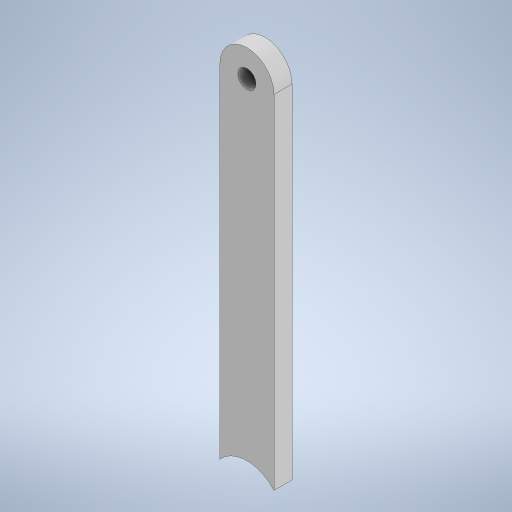
# Autodesk Inventor part: Conn Rod Rod Portion
Saved by Autodesk Inventor 2023 (Build 270158000, 158)
## iProperties
Created: 2023-02-24
Part Number: Conn Rod Rod Portion
Material: Generic
Document SubType Name: Modeling
Designer: tommy
Density: 1 g/cm^3
Appearance: Default
Author: tommy
Autodesk Inventor part; units mm, degrees
ref_plane "YZ Plane" through (0, 0, 0) normal (1, 0, 0) x (0, 1, 0)
ref_plane "XZ Plane" through (0, 0, 0) normal (0, 1, 0) x (-1, 0, 0)
ref_plane "XY Plane" through (0, 0, 0) normal (0, 0, 1) x (1, 0, 0)
sketch "Sketch1" plane through (0, 0, 0) normal (0, 0, 1) x (1, 0, 0)
  circle A0 centre (1.1906, -1.1906) radius 0.3969
  arc A1 (2.3813, -1.1906) -> (0, -1.1906) centre (1.1906, -1.1906) ccw
  line L0 (1.1906, -1.1906) -> (1.1906, 0)
  line L1 (0, 0) -> (0, -17.3482)
  line L2 (0, -17.3482) -> (2.3813, -17.3482)
  line L3 (2.3813, -17.3482) -> (2.3813, -1.1906)
  circle A2 centre (1.1906, -17.3482) radius 1.5875
  point P0 (1.1906, 0)
  point P1 (0, -1.1906)
  point P2 (0, -16.2982)
  point P3 (2.3813, -16.2982)
  dimension "d4" = 17.3482
  dimension "d5" = 3.175
  constraints: 8 end point, 4 point on circle, 3 centre point, 2 perpendicular, 2 vertical, 1 coincident, 1 midpoint
  measures "d4" distance of L1.start L1.end
  measures "d5" diameter of A2
extrude "Extrusion1" add sketch "Sketch1" along normal blind 0.7937 contours L3 A2 L1 A1
body "Solid1"
